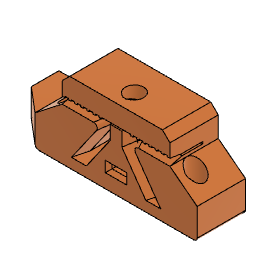
y_belt_holder_9mm_belt_bear2.1_mk2s-2.5-2.5s (Autodesk Fusion 360 archive; units mm, degrees)
design "y_belt_holder"
Autodesk Fusion 360 part; units mm, degrees
sketch "Sketch1" plane through (0, 0, 0) normal (0, 0, 1) x (1, 0, 0) in component "y_belt_holder"
  line L0 (-14, 10.3) -> (47, 10.3)
  line L1 (47, 10.3) -> (47, -5.5)
  line L2 (47, -5.5) -> (-14, -5.5)
  line L3 (-14, -5.5) -> (-14, 10.3)
  circle A0 centre (0, 0) radius 1.65
  circle A1 centre (41, 0) radius 1.65
  line L4 (0, 0) -> (41, 0) construction
  line L5 (2.9, 10.3) -> (2.9, -5.5)
  line L6 (38.1, 10.3) -> (38.1, -5.5)
  circle A2 centre (0, 0) radius 2.9
  circle A3 centre (41, 0) radius 2.9
  line L7 (0.825, -1.4289) -> (0.0957, -1.85)
  line L8 (0.0957, -1.85) -> (-0.0957, -1.85)
  line L9 (-0.0957, -1.85) -> (-0.825, -1.4289)
  line L10 (1.45, -2.5115) -> (0.4306, -3.1)
  line L11 (0.4306, -3.1) -> (-0.4306, -3.1)
  line L12 (-0.4306, -3.1) -> (-1.45, -2.5115)
  line L13 (41.825, -1.4289) -> (41.0957, -1.85)
  line L14 (41.0957, -1.85) -> (40.9043, -1.85)
  line L15 (40.9043, -1.85) -> (40.175, -1.4289)
  line L16 (42.45, -2.5115) -> (41.4306, -3.1)
  line L17 (41.4306, -3.1) -> (40.5694, -3.1)
  line L18 (40.5694, -3.1) -> (39.55, -2.5115)
  circle A4 centre (20.5, 0) radius 1.65
  circle A5 centre (20.5, 0) radius 3
  circle A6 centre (20.5, 0) radius 3.1 construction
  line L19 (20.5, -3.1) -> (23.1847, -1.55)
  line L20 (23.1847, -1.55) -> (23.1847, 1.55)
  line L21 (23.1847, 1.55) -> (20.5, 3.1)
  line L22 (20.5, 3.1) -> (17.8153, 1.55)
  line L23 (17.8153, 1.55) -> (17.8153, -1.55)
  line L24 (17.8153, -1.55) -> (20.5, -3.1)
  line L25 (-14, 5.5) -> (47, 5.5) construction
  line L26 (-14, -0.5) -> (47, -0.5) construction
  line L27 (19.675, -1.4289) -> (20.4043, -1.85)
  line L28 (20.4043, -1.85) -> (20.5957, -1.85)
  line L29 (20.5957, -1.85) -> (21.325, -1.4289)
  line L30 (19, -2.5981) -> (20.0426, -3.2)
  line L31 (20.0426, -3.2) -> (20.9574, -3.2)
  line L32 (20.9574, -3.2) -> (22, -2.5981)
  line L33 (-14, 1.3) -> (-6, -5.5)
  point P0 (20.5, 0)
  dimension "d2" = 3.3
  dimension "d3" = 3.3
  dimension "d4" = 41
  dimension "d5" = 14
  dimension "d8" = 5.8
  dimension "d9" = 5.8
  dimension "d11" = 5.5
  dimension "d58" = 150
  dimension "d60" = 150
  dimension "d62" = 150
  dimension "d64" = 150
  dimension "d67" = 150
  dimension "d68" = 150
  dimension "d69" = 150
  dimension "d70" = 150
  dimension "d71" = 0.2
  dimension "d72" = 0.2
  dimension "d73" = 0.2
  dimension "d74" = 0.2
  dimension "d83" = 6
  dimension "d157" = 6
  dimension "d158" = 3.3
  dimension "d160" = 6.2
  dimension "d218" = 5.5
  dimension "d219" = 6
  dimension "d220" = 4.8
  dimension "d273" = 150
  dimension "d274" = 0.2
  dimension "d275" = 150
  dimension "d276" = 150
  dimension "d277" = 150
  dimension "d278" = 0.2
  dimension "d367" = 9
  dimension "d369" = 6
  dimension "d370" = 44.275
  constraint horizontal L0
  constraint vertical L1
  constraint horizontal L2
  constraint vertical L3
  constraint coincident A0.centre L4.start
  constraint coincident A1.centre L4.end
  constraint horizontal L4
  constraint coincident L0 L5.start
  constraint coincident L2 L5.end
  constraint perpendicular L2 L5
  constraint coincident L0 L6.start
  constraint coincident L2 L6.end
  constraint perpendicular L2 L6
  constraint concentric A0 A2
  constraint concentric A1 A3
  constraint coincident A0 L7.start
  constraint tangent A0 L7
  constraint coincident A0 L9.end
  constraint tangent A0 L9
  constraint coincident A2 L10.start
  constraint tangent A2 L10
  constraint parallel L8 L11
  constraint coincident A2 L12.end
  constraint tangent A2 L12
  constraint coincident A1 L13.start
  constraint tangent A1 L13
  constraint coincident A1 L15.end
  constraint tangent A1 L15
  constraint coincident A3 L16.start
  constraint tangent A3 L16
  constraint parallel L14 L17
  constraint coincident A3 L18.end
  constraint tangent A3 L18
  constraint horizontal L11
  constraint horizontal L17
  constraint tangent L5 A2
  constraint tangent L6 A3
  constraint concentric A4 A5
  constraint concentric A4 A6
  constraint coincident A6 L19.start
  constraint coincident P0 A4.centre
  constraint vertical L23
  constraint coincident L3 L25.start
  constraint coincident L1 L25.end
  constraint perpendicular L1 L25
  constraint coincident L3 L26.start
  constraint coincident L1 L26.end
  constraint perpendicular L1 L26
  constraint coincident A4 L27.start
  constraint horizontal L28
  constraint coincident A4 L29.end
  constraint coincident A5 L30.start
  constraint tangent A5 L30
  constraint parallel L28 L31
  constraint coincident A5 L32.end
  constraint tangent A5 L32
  constraint tangent A4 L27
  constraint tangent A4 L29
  constraint midpoint L4 P0
  constraint coincident L3 L33.start
  constraint coincident L2 L33.end
  measures "d2" diameter of A0
  measures "d3" diameter of A1
  measures "d4" distance of A0.centre A1.centre
  measures "d5" distance of A0.centre L3
  measures "d8" diameter of A2
  measures "d9" diameter of A3
  measures "d11" vertical distance of L2.end A0.centre
  measures "d58" angle of L7 L8
  measures "d60" angle of L8 L9
  measures "d62" angle of L10 L11
  measures "d64" angle of L11 L12
  measures "d67" angle of L16 L17
  measures "d68" angle of L17 L18
  measures "d69" angle of L13 L14
  measures "d70" angle of L14 L15
  measures "d71" distance of A2 L11
  measures "d72" distance of A0 L8
  measures "d73" distance of A3 L17
  measures "d74" distance of A1 L14
  measures "d83" distance of L1 A1.centre
  measures "d157" diameter of A5
  measures "d158" diameter of A4
  measures "d160" diameter of A6
  measures "d218" vertical distance of A0.centre L25.start
  measures "d219" distance of L25 L26
  measures "d220" distance of L0 L25.start
  measures "d273" angle of L27 L28
  measures "d274" distance of A4 L28
  measures "d275" angle of L28 L29
  measures "d276" angle of L30 L31
  measures "d277" angle of L31 L32
  measures "d278" distance of A5 L31
  measures "d367" distance of L0.start L33.start
  measures "d369" horizontal distance of A0.centre L33.end
extrude "Extrude1" add sketch "Sketch1" along normal blind 26 contours L0 L2 L5 L6 | A4 | A4 L27 L28 L29 | A5 L20 | A5 L19 L20 L21 L22 L23 L24 | A5 L20 L21 | A5 L19 L20 | A5 L21 | A5 L19 | A5 L21 L22 | A5 L19 L24 L30 L31 L32 | A5 L19 L24 | A5 L22 | A5 L24 | A5 L22 L23 | A5 L23 L24 | A5 L23 in component "y_belt_holder"
extrude "Extrude2" add sketch "Sketch1" along normal blind 10 contours A2 | L0 L2 L3 L5 L33 | A3 | L0 L1 L2 L6 | A2 L10 L11 L12 | A3 L16 L17 L18 | A0 | A0 L7 L8 L9 | A1 | A1 L13 L14 L15 in component "y_belt_holder"
extrude "Extrude11" cut sketch "Sketch1" along normal blind 39 contours A4 | A4 L27 L28 L29 in component "y_belt_holder"
sketch "Sketch2" plane through (0, -5.5, 0) normal (0, -1, 0) x (1, 0, 0) in component "y_belt_holder"
  line L0 (-6, 0) -> (47, 0)
  line L1 (47, 0) -> (47, 10)
  line L2 (47, 10) -> (38.1, 10)
  line L3 (38.1, 10) -> (38.1, 26)
  line L4 (38.1, 26) -> (2.9, 26)
  line L5 (2.9, 26) -> (2.9, 10)
  line L6 (38.1, 17.9) -> (26.5535, 17.9)
  line L7 (2.9, 17.9) -> (14.4465, 17.9)
  line L8 (2.9, 19.55) -> (38.1, 19.55)
  line L9 (20.5, 26) -> (20.5, 0) construction
  arc A0 (26.5535, 17.9) -> (25.3247, 15.5396) centre (26.5535, 16.4) ccw
  line L10 (22.15, 26) -> (22.15, 7.35) construction
  line L11 (18.85, 26) -> (18.85, 7.35) construction
  line L12 (25.3247, 15.5396) -> (33.8652, 3.3426)
  line L13 (23.4035, 14.7966) -> (31.4237, 3.3426)
  line L14 (31.4237, 3.3426) -> (33.8652, 3.3426)
  arc A1 (15.6753, 15.5396) -> (14.4465, 17.9) centre (14.4465, 16.4) ccw
  line L15 (17.5965, 14.7966) -> (9.5763, 3.3426)
  line L16 (9.5763, 3.3426) -> (7.1348, 3.3426)
  line L17 (7.1348, 3.3426) -> (15.6753, 15.5396)
  line L18 (2.9, 18.55) -> (3.8, 18.55)
  line L19 (3.8, 18.55) -> (3.8, 19.55)
  line L20 (17.5965, 19.05) -> (23.4035, 19.05)
  line L21 (23.4035, 19.05) -> (23.4035, 14.7966)
  line L22 (38.1, 19.55) -> (38.1, 18.55)
  line L23 (38.1, 18.55) -> (37.2, 18.55)
  line L24 (37.2, 18.55) -> (37.2, 19.55)
  line L25 (4.9, 19.55) -> (4.9, 18.55)
  line L26 (4.9, 18.55) -> (5.8, 18.55)
  line L27 (5.8, 18.55) -> (5.8, 19.55)
  line L28 (35.2, 19.55) -> (35.2, 18.55)
  line L29 (35.2, 18.55) -> (36.1, 18.55)
  line L30 (36.1, 18.55) -> (36.1, 19.55)
  line L31 (6.9, 19.55) -> (6.9, 18.55)
  line L32 (7.8, 18.55) -> (7.8, 19.55)
  line L33 (6.9, 18.55) -> (7.8, 18.55)
  line L34 (8.9, 19.55) -> (8.9, 18.55)
  line L35 (9.8, 18.55) -> (9.8, 19.55)
  line L36 (8.9, 18.55) -> (9.8, 18.55)
  line L37 (10.9, 19.55) -> (10.9, 18.55)
  line L38 (11.8, 18.55) -> (11.8, 19.55)
  line L39 (10.9, 18.55) -> (11.8, 18.55)
  line L40 (12.9, 19.55) -> (12.9, 18.55)
  line L41 (13.8, 18.55) -> (13.8, 19.55)
  line L42 (12.9, 18.55) -> (13.8, 18.55)
  line L43 (14.9, 19.55) -> (14.9, 18.55)
  line L44 (15.8, 18.55) -> (15.8, 19.55)
  line L45 (14.9, 18.55) -> (15.8, 18.55)
  line L46 (33.2, 18.55) -> (34.1, 18.55)
  line L47 (34.1, 18.55) -> (34.1, 19.55)
  line L48 (33.2, 19.55) -> (33.2, 18.55)
  line L49 (31.2, 18.55) -> (32.1, 18.55)
  line L50 (32.1, 18.55) -> (32.1, 19.55)
  line L51 (31.2, 19.55) -> (31.2, 18.55)
  line L52 (29.2, 18.55) -> (30.1, 18.55)
  line L53 (30.1, 18.55) -> (30.1, 19.55)
  line L54 (29.2, 19.55) -> (29.2, 18.55)
  line L55 (27.2, 18.55) -> (28.1, 18.55)
  line L56 (28.1, 18.55) -> (28.1, 19.55)
  line L57 (27.2, 19.55) -> (27.2, 18.55)
  line L58 (25.2, 18.55) -> (26.1, 18.55)
  line L59 (26.1, 18.55) -> (26.1, 19.55)
  line L60 (25.2, 19.55) -> (25.2, 18.55)
  line L61 (17.5965, 14.7966) -> (17.5965, 19.05)
  line L62 (18.85, 26) -> (22.15, 26)
  line L63 (17.5965, 17.9) -> (23.4035, 17.9)
  line L64 (18.85, 16.5867) -> (7.2358, 0) construction
  line L65 (2.9, 16.9) -> (-6, 10)
  line L66 (38.1, 16.9) -> (47, 10)
  line L67 (17.7, 7.35) -> (23.3, 7.35)
  line L68 (23.3, 7.35) -> (23.3, 5.25)
  line L69 (23.3, 5.25) -> (17.7, 5.25)
  line L70 (17.7, 5.25) -> (17.7, 7.35)
  line L71 (35.65, 26) -> (38.1, 23.55)
  line L72 (2.9, 23.55) -> (5.35, 26)
  line L73 (2.9, 10) -> (-6, 10)
  line L74 (-6, 10) -> (-6, 0)
  point P0 (41, 0)
  dimension "d185" = 0.9
  dimension "d190" = 1.5
  dimension "d191" = 1.5
  dimension "d205" = 0.9
  dimension "d206" = 0.9
  dimension "d207" = 2
  dimension "d211" = 0.9
  dimension "d212" = 2
  dimension "d224" = 2
  dimension "d225" = 0
  dimension "d228" = 2
  dimension "d229" = 0
  dimension "d230" = 1.2535
  dimension "d232" = 1.2535
  dimension "d233" = 0.5
  dimension "d235" = 1.65
  dimension "d238" = 1.65
  dimension "d263" = 2
  dimension "d265" = 2
  dimension "d266" = 3.3426
  dimension "d284" = 1
  dimension "d327" = 2.1
  dimension "d328" = 5.6
  dimension "d355" = 1
  dimension "d356" = 7.9
  dimension "d357" = 1.65
  dimension "d358" = 1
  dimension "d359" = 55
  dimension "d362" = 45
  dimension "d364" = 4
  dimension "d372" = 12.2
  constraint perpendicular L3 L6
  constraint coincident L3 L8.end
  constraint perpendicular L5 L7
  constraint coincident L5 L8.start
  constraint perpendicular L5 L8
  constraint midpoint L4 L9.start
  constraint coincident L0 L9.end
  constraint tangent L6 A0
  constraint tangent A0 L12
  constraint tangent L7 A1
  constraint tangent A1 L17
  constraint coincident L5 L18.start
  constraint perpendicular L5 L18
  constraint coincident L8 L19.end
  constraint perpendicular L8 L19
  constraint perpendicular L9 L20
  constraint perpendicular L20 L21
  constraint coincident L3 L22.end
  constraint perpendicular L22 L23
  constraint coincident L8 L25.start
  constraint perpendicular L8 L25
  constraint perpendicular L25 L26
  constraint coincident L8 L27.end
  constraint perpendicular L8 L27
  constraint collinear L18 L26
  constraint perpendicular L28 L29
  constraint collinear L23 L29
  constraint vertical L61
  constraint coincident L15.start L61.start
  constraint coincident L13.start L21.end
  constraint coincident L11.start L62.start
  constraint coincident L10.start L62.end
  constraint coincident L61 L63.start
  constraint coincident L21 L63.end
  constraint perpendicular L21 L63
  constraint collinear L7 L63
  constraint parallel L0 L14
  constraint parallel L0 L16
  constraint parallel L12 L13
  constraint parallel L15 L17
  constraint collinear L14 L16
  constraint coincident L11 L64.start
  constraint coincident L0 L64.end
  constraint parallel L15 L64
  constraint horizontal L67
  constraint vertical L68
  constraint horizontal L69
  constraint vertical L70
  constraint symmetric L9 L68 L70
  constraint coincident L11.end L67
  constraint coincident L10.end L67
  constraint coincident L3 L6.start
  constraint coincident L3 L66.start
  constraint coincident L8.end L22.start
  constraint coincident L8 L24.end
  constraint coincident L8 L30.end
  constraint coincident L8 L28.start
  constraint collinear L18 L23
  constraint coincident L5 L65.start
  constraint coincident L5 L7.start
  constraint collinear L6 L7
  constraint symmetric L9 L65 L66
  constraint coincident L4 L71.start
  constraint coincident L3 L71.end
  constraint coincident L5 L72.start
  constraint coincident L4 L72.end
  constraint symmetric L9 L71 L72
  constraint coincident L1.end L2.start
  constraint coincident L65.end L73.end
  measures "d185" distance of L8.start L19
  measures "d190" radius of A1
  measures "d191" radius of A0
  measures "d205" distance of L22 L24
  measures "d206" distance of L25 L27
  measures "d207" distance of L8.start L25
  measures "d211" distance of L28 L30
  measures "d212" distance of L22 L30
  measures "d230" distance of L10 L21
  measures "d232" distance of L11 L61
  measures "d233" distance of L8 L20
  measures "d235" distance of A1 L61
  measures "d238" distance of A0 L21
  measures "d263" distance of L15 L17
  measures "d265" distance of L12 L13
  measures "d266" distance of L0 L16
  measures "d284" distance of L8 L18
  measures "d327" distance of L67.start L69.end
  measures "d328" distance of L68.end L69.end
  measures "d355" distance of L66.start L6.start
  measures "d356" distance of L5.end L7.start
  measures "d357" distance of L8.start L7.start
  measures "d358" distance of L65.start L7.start
  measures "d359" angle of L6 L12
  measures "d362" angle of L4 L71
  measures "d364" distance of L8.end L71.end
  measures "d372" vertical distance of L8.start L67.start
extrude "Extrude10" cut sketch "Sketch2" against normal up to surface (10.7 mm away) contours L3 L5 L6 L7 L8 A0 L12 L13 L14 A1 L15 L16 L17 L18 L19 L20 L21 L23 L24 L25 L26 L27 L28 L29 L30 L31 L32 L33 L34 L35 L36 L37 L38 L39 L40 L41 L42 L43 L44 L45 L46 L47 L48 L49 L50 L51 L52 L53 L54 L55 L56 L57 L58 L59 L60 L61 in component "y_belt_holder"
extrude "Extrude1'" cut sketch "Sketch2" against normal blind 8.5 contours L67 L68 L69 L70 in component "y_belt_holder"
extrude "Extrude18" cut sketch "Sketch2" along normal blind 1.15 from surface at -10.7 contours L20 L21 L61 L63 in component "y_belt_holder"
draft "Draft1" angle 45 neutral plane through (17.5965, -5.5, 19.05) pull (0, 0, 1) 1 faces at (19.5322, 4.05, 18.6667) in component "y_belt_holder"
move_face "OffsetFaces1" offset -0.1 4 faces at (21.4632, -1.3397, 21.7) (19.9181, -1.5693, 21.7) (21.0819, -1.5693, 21.7) (20.4681, -1.85, 23.85) in component "y_belt_holder"
fillet "Fillet2" radius 1 2 edges at (23.4035, -0.725, 19.05) (17.5965, -0.725, 19.05) in component "y_belt_holder"
extrude "Extrude23" add sketch "Sketch2" against normal up to surface (15.8 mm away) contours L5 L65 L73 | L2 L3 L66 in component "y_belt_holder"
extrude "Extrude3" cut sketch "Sketch2" against normal up to surface (15.8 mm away) contours L4 L5 L72 | L3 L4 L71 in component "y_belt_holder"
extrude "Extrude5" cut sketch "Sketch1" along normal blind 21 contours A2 | A3 | A2 L10 L11 L12 | A3 L16 L17 L18 | A0 | A0 L7 L8 L9 | A1 | A1 L13 L14 L15 in component "y_belt_holder"
extrude "Extrude6" add sketch "Sketch1" along normal blind 4 contours A2 | A3 | A2 L10 L11 L12 | A3 L16 L17 L18 in component "y_belt_holder"
fillet "Fillet4" radius 0.6 12 edges at (-0.4604, -1.6395, 0) (0, 1.65, 0) (0.4604, -1.6395, 0) (0, -1.85, 0) (41, -1.85, 0) (40.5396, -1.6395, 0) (41, 1.65, 0) (41.4604, -1.6395, 0) (20.9604, -1.6395, 0) (20.5, 1.65, 0) (20.0396, -1.6395, 0) (20.5, -1.85, 0) in component "y_belt_holder"
chamfer "Chamfer8" distance 0.5 angle 45 1 edges at (16.5, 10.3, 0) in component "y_belt_holder"
fillet "Fillet5" radius 1 3 edges at (-14, 5.55, 0) (47, 2.15, 0) (-10, -2.1, 0) in component "y_belt_holder"
sketch "Sketch5" plane through (38.1, 0, 0) normal (1, 0, 0) x (0, 1, 0) in component "y_belt_holder"
  line L0 (-5.5, 17.9) -> (-5.5, 16.9)
  line L1 (-5.5, 18.55) -> (5.2, 18.55)
  line L2 (5.2, 18.55) -> (5.2, 17.9)
  line L3 (10.3, 16.9) -> (10.3, 23.55)
  line L4 (-5.5, 18.55) -> (5.2, 18.55)
  line L5 (-5.5, 18.55) -> (-5.5, 23.55)
  line L6 (5.2, 18.55) -> (-5.5, 18.55)
  line L7 (-5.5, 19.15) -> (-1.4, 18.55)
  line L8 (0, 16.9) -> (10.3, 16.9)
  line L9 (-5.5, 23.55) -> (-5.5, 18.55)
  line L10 (-5.5, 19.55) -> (5.2, 19.55)
  dimension "d365" = 6.6
  dimension "d366" = 0.4
  constraint coincident L6 L7.end
  constraint coincident L5 L7.start
  measures "d365" distance of L1.end L7.end
  measures "d366" distance of L7.start L10.start
extrude "Extrude15" cut sketch "Sketch5" against normal up to surface (14.6965 mm away) in component "y_belt_holder"
extrude "Extrude16" cut sketch "Sketch5" along normal up to surface (14.6965 mm away) from surface at -35.2 in component "y_belt_holder"
chamfer "Chamfer6" distance 1 distance2 4 6 edges at (13.5864, -5.5, 9.0696) (17.5965, -5.5, 16.4233) (23.4035, -5.5, 16.4233) (27.4136, -5.5, 9.0696) (32.3267, -5.5, 17.9) (8.6733, -5.5, 17.9) measured on face at (32.43, -5.5, 11.9274) measured on face at (32.43, -5.5, 11.9274) measured on face at (32.43, -5.5, 11.9274) measured on face at (32.43, -5.5, 11.9274) measured on face at (32.43, -5.5, 11.9274) measured on face at (32.43, -5.5, 11.9274) tangent chain off in component "y_belt_holder"
chamfer "Chamfer7" distance 1 distance2 5 2 edges at (11.405, -5.5, 9.4411) (29.595, -5.5, 9.4411) measured on face at (32.43, -5.5, 11.9274) measured on face at (32.43, -5.5, 11.9274) tangent chain off in component "y_belt_holder"
fillet "Fillet3" radius 1.2 2 edges at (25.4136, -5.0721, 17.007) (15.5864, -5.0721, 17.007) in component "y_belt_holder"
ref_plane "WorkPlane3" through (20.5, 2.4, 13) normal (1, 0, 0) x (0, 1, 0) in component "y_belt_holder"
chamfer "Chamfer1" distance 0.7 distance2 1.5 4 edges at (20.5, -5.5, 5.25) (20.5, -5.5, 7.35) (17.7, -5.5, 6.3) (23.3, -5.5, 6.3) measured on face at (33.3588, -5.5, 11.7632) measured on face at (33.3588, -5.5, 11.7632) measured on face at (33.3588, -5.5, 11.7632) measured on face at (33.3588, -5.5, 11.7632) in component "y_belt_holder"
sketch "Sketch10" plane through (20.5, 2.7, 18.5) normal (1, 0, 0) x (0, 1, 0) in component "y_belt_holder"
  line L0 (-8.2, 1.05) -> (2.5, 1.05)
  line L1 (-8.2, 1.05) -> (2.5, -0.6) construction
  line L2 (-2.7, -18.5) -> (-2.7, 4.15) construction
  line L3 (-8.2, 0.65) -> (-8.2, 5.05)
  line L4 (7.6, -1.6) -> (7.6, 5.05)
  line L5 (-8.2, 4.9981) -> (7.6, 2.5617)
  line L6 (-6.7, -11.15) -> (0.3, -11.15)
  line L7 (-8.2, 5.05) -> (-8.2, 7.5)
  point P0 (2.5, -0.6)
  point P1 (-2.7, -18.5)
  dimension "d336" = 15.3
  constraint coincident L0.start L1.start
  constraint coincident P0 L1.end
  constraint vertical L2
  constraint coincident L4 L5.end
  constraint coincident L2.end L5
  constraint parallel L1 L5
  constraint coincident P1 L2.start
  constraint coincident L3 L5.start
  measures "d336" distance of L2.end L6
ref_plane "WorkPlane4" through (20.5, 2.4, 22.2799) normal (0, 0.152404, 0.988318) x (0, 0.988318, -0.152404) in component "y_belt_holder"
sketch "Sketch11" plane through (20.5, 2.4452, 22.2729) normal (0, 0.152404, 0.988318) x (0, 0.988318, -0.152404) in component "y_belt_holder"
  circle A0 centre (-2.4741, 0) radius 3
  line L0 (-5.0722, -1.5) -> (-5.6741, -0.4574)
  line L1 (-5.6741, -0.4574) -> (-5.6741, 0.4574)
  line L2 (-5.6741, 0.4574) -> (-5.0722, 1.5)
  point P0 (-2.4741, 0)
  dimension "d317" = 6
  dimension "d320" = 0.2
  dimension "d321" = 150
  dimension "d322" = 150
  constraint coincident P0 A0.centre
  constraint coincident A0 L0.start
  constraint tangent A0 L0
  constraint vertical L1
  constraint coincident A0 L2.end
  constraint tangent A0 L2
  measures "d317" diameter of A0
  measures "d320" distance of A0 L1
  measures "d321" angle of L1 L2
  measures "d322" angle of L0 L1
extrude "Extrude22" cut sketch "Sketch11" along normal blind 7 in component "y_belt_holder"
ref_plane "WorkPlane2" through (20.5, 0, 0) normal (0, 1, 0) x (1, 0, 0) in component "y_belt_holder"
sketch "Sketch9" plane through (20.5, 0, 0) normal (0, 1, 0) x (1, 0, 0) in component "y_belt_holder"
  line L0 (-2.9035, -14.7966) -> (-10.9237, -3.3426)
  line L1 (-1.65, -19.05) -> (1.65, -19.05)
  line L2 (-1.65, -7.35) -> (-1.65, -19.05) construction
  line L3 (-3.4223, -9.9365) -> (-3.3213, -9.9365)
  line L4 (-3.3213, -9.9365) -> (-3.3213, -9.8355)
  line L5 (-3.3213, -9.8355) -> (-3.4223, -9.8355)
  line L6 (-3.4223, -9.8355) -> (-3.4223, -9.9365)
  line L7 (1.65, -7.35) -> (-1.65, -7.35)
  line L8 (-2.8, -5.25) -> (-2.8, -7.35)
  line L9 (-5.2855, -7.0614) -> (-5.3865, -6.9171)
  line L10 (-5.3865, -6.9171) -> (-5.3865, -5.25)
  line L11 (-5.3865, -5.25) -> (-5.2855, -5.25)
  line L12 (-5.2855, -5.25) -> (-5.2855, -7.0614)
  line L13 (10.9237, -3.3426) -> (2.9035, -14.7966)
  line L14 (2.8, -7.35) -> (2.8, -5.25)
  line L15 (-2.8, -5.25) -> (-5.2855, -5.25) construction
  line L16 (5.3865, -6.9171) -> (5.2855, -7.0614)
  line L17 (5.2855, -7.0614) -> (5.2855, -5.25)
  line L18 (5.2855, -5.25) -> (5.3865, -5.25)
  line L19 (5.3865, -5.25) -> (5.3865, -6.9171)
  line L20 (5.2855, -5.25) -> (2.8, -5.25) construction
  line L21 (0, -19.05) -> (0, -7.35) construction
  line L22 (3.4223, -9.8355) -> (3.4223, -9.9365)
  line L23 (3.4223, -9.9365) -> (3.3213, -9.9365)
  line L24 (3.3213, -9.8355) -> (3.4223, -9.8355)
  line L25 (3.3213, -9.9365) -> (3.3213, -9.8355)
  dimension "d306" = 1.6713
  dimension "d308" = 0.101
  dimension "d309" = 0.101
  dimension "d337" = 2.4855
  dimension "d338" = 2.4855
  dimension "d340" = 0.101
  dimension "d344" = 2.4855
  dimension "d345" = 2.4855
  dimension "d346" = 0.101
  dimension "d347" = 2.4855
  constraint coincident L1.start L2.end
  constraint horizontal L3
  constraint vertical L4
  constraint horizontal L5
  constraint vertical L6
  constraint coincident L2.start L7.end
  constraint vertical L10
  constraint horizontal L11
  constraint vertical L12
  constraint parallel L0 L9
  constraint coincident L8.start L15.start
  constraint horizontal L15
  constraint vertical L17
  constraint horizontal L18
  constraint vertical L19
  constraint parallel L13 L16
  constraint coincident L14.end L20.end
  constraint horizontal L20
  constraint midpoint L1 L21.start
  constraint midpoint L7 L21.end
  constraint symmetric L3.start L21 L22.end
  constraint symmetric L3.end L21 L23.end
  constraint symmetric L4.end L21 L24.start
  constraint symmetric L5.end L21 L22.start
  measures "d306" distance of L2 L4
  measures "d308" distance of L4.end L5.end
  measures "d309" distance of L3.end L4.end
  measures "d337" distance of L5 L7
  measures "d338" distance of L8 L12
  measures "d340" distance of L10 L12
  measures "d344" distance of L14 L17
  measures "d345" distance of L13 L16
  measures "d346" distance of L17.end L18.end
  measures "d347" distance of L0 L9
extrude "Extrude21" cut sketch "Sketch9" along normal mid plane 0.4 contours L3 L4 L5 L6 | L22 L23 L24 L25 in component "y_belt_holder"
extrude "Extrude2'" cut sketch "Sketch9" against normal up to surface (6.5 mm away) from surface at 3 contours L9 L10 L11 L12 | L16 L17 L18 L19 in component "y_belt_holder"
move_body "Move1" [suppressed] in component "y_belt_holder"
component "y_belt_holder" placed x (1, 0, 0) y (0, 1, 0) z (0, 0, 1) at (0, 0, 0)
equation "m3_hole = 3.3 mm"
equation "d2 = m3_hole"
equation "d3 = m3_hole"
equation "m3_head = 5.8 mm"
equation "d8 = m3_head"
equation "d9 = m3_head"
equation "layer_height = 0.2 mm"
equation "d71 = layer_height"
equation "d72 = layer_height"
equation "d73 = layer_height"
equation "d74 = layer_height"
equation "extrusion_width = 0.45 mm"
equation "num_perimeters = 4"
equation "num_top_bottoms = 5"
equation "top_bottom_thickness = num_top_bottoms * layer_height"
equation "perimeters_width = extrusion_width + ( num_perimeters - 1 ) * 0.4071 mm"
equation "d157 = m3_head + 0.2 mm"
equation "d158 = m3_hole"
equation "m3_nut = 6.2 mm"
equation "d160 = m3_nut"
equation "belt_path_thickness = 1.65 mm"
equation "d198 = -back_thickness - 0.3 mm"
equation "d206 = d185"
equation "d220 = back_thickness"
equation "back_thickness = 4.8 mm"
equation "d230 = perimeters_width * 3 / 4"
equation "d232 = perimeters_width * 3 / 4"
equation "d233 = flex_opening"
equation "d235 = belt_path_thickness"
equation "d238 = belt_path_thickness"
equation "d266 = perimeters_width * 2"
equation "d269 = belt_path_thickness - flex_opening"
equation "d274 = layer_height"
equation "d275 = d273"
equation "d277 = d276"
equation "d278 = layer_height"
equation "d284 = belt_teeth_height"
equation "belt_teeth_height = 1 mm"
equation "flex_opening = 0.5 mm"
equation "d302 = layer_height * 2"
equation "d306 = perimeters_width"
equation "d317 = m3_head + 0.2 mm"
equation "d320 = layer_height"
equation "d332 = -5.5 mm - 3 mm"
equation "d337 = extrusion_width + 5 * 0.4071 mm"
equation "d338 = extrusion_width + 5 * 0.4071 mm"
equation "d342 = -top_bottom_thickness * 2"
equation "d344 = extrusion_width + 5 * 0.4071 mm"
equation "d345 = extrusion_width + 5 * 0.4071 mm"
equation "d347 = extrusion_width + 5 * 0.4071 mm"
equation "d357 = belt_path_thickness"
equation "d369 = d83"
